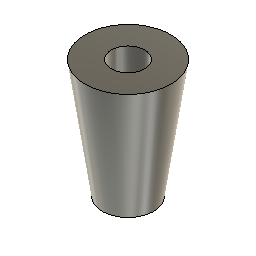
xy_Right_9mm_Pinned_Lower_Final v25 (Autodesk Fusion 360 archive; units mm, degrees)
design "Hole support"
Autodesk Fusion 360 part; units mm, degrees
sketch "Sketch1" plane through (0, 0, 0) normal (1, 0, 0) x (0, 1, 0)
  line L0 (0, 0) -> (2.7, 0) construction
  line L1 (2.7, 0) -> (2.7, 19.4)
  line L2 (2.7, 19.4) -> (7, 19.4)
  line L3 (2.7, 0) -> (4.2, 0)
  line L4 (7, 19.4) -> (4.2, 0)
  dimension "d1" = 2.7
  dimension "d2" = 19.4
  dimension "d3" = 4.3
  dimension "d5" = 1.5
  constraint coincident L0.start origin
  constraint horizontal L0
  constraint perpendicular L0 L1
  constraint perpendicular L1 L2
  constraint perpendicular L1 L3
  measures "d1" distance of L0.start L0.end
  measures "d2" distance of L0.end L1.end
  measures "d3" distance of L1.end L2.end
  measures "d5" distance of L0.end L3.end
revolve "Revolve1" add sketch "Sketch1" angle 360 about axis through (0, 0, 1.75) along (0, 0, 1)
